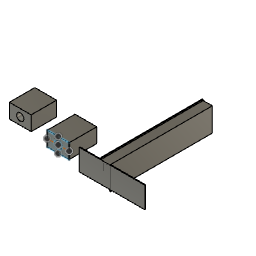
WhiteBoardMount v10 (Autodesk Fusion 360 design; units mm, degrees)
Autodesk Fusion 360 part; units mm, degrees
sketch "Sketch1" plane through (0, 0, 0) normal (0, 1, 0) x (1, 0, 0) in component "Mount"
  line L0 (0, 0) -> (-4.6, 0)
  line L1 (0, 0) -> (0, 30)
  line L2 (0, 30) -> (2, 30)
  line L3 (2, 30) -> (2, -4)
  line L4 (-4.6, 0) -> (-4.6, 10)
  line L5 (-4.6, 10) -> (-6.6, 10)
  line L6 (-6.6, 10) -> (-6.6, 0)
  line L7 (-6.6, 0) -> (-11.6, 0)
  line L8 (-11.6, 0) -> (-11.6, -4)
  line L9 (-11.6, -4) -> (2, -4)
  line L10 (-11.6, -4) -> (-10.6, -4)
  line L11 (-10.6, -4) -> (-10.6, -4)
  line L12 (-10.6, -4) -> (-11.6, -4)
  line L13 (-11.6, -4) -> (-11.6, -4)
  line L14 (-10.6, -4) -> (-10.6, -2.5)
  line L15 (2, -2.5) -> (1, -2.5) construction
  line L16 (-10.6, -2.5) -> (2, -2.5)
  line L17 (50.1972, -2.5) -> (-40, -2.5)
  line L18 (-40, -2.5) -> (-40, 0)
  line L19 (-40, 0) -> (50.1972, 0)
  line L20 (50.1972, 0) -> (50.1972, -2.5)
  line L21 (50, 23.4656) -> (-40, 23.4656)
  line L22 (-40, 23.4656) -> (-40, 21.2216)
  line L23 (-40, 21.2216) -> (50, 21.2216)
  line L24 (50, 21.2216) -> (50, 23.4656)
  dimension "d1" = 4.6
  dimension "d2" = 30
  dimension "d3" = 2
  dimension "d4" = 34
  dimension "d5" = 2
  dimension "d6" = 10
  dimension "d7" = 10
  dimension "d8" = 5
  dimension "d9" = 4
  dimension "d14" = 1
  dimension "d15" = 1.5
  dimension "d16" = 1
  constraint coincident L0.start L1.start
  constraint horizontal L0
  constraint perpendicular L0 L1
  constraint perpendicular L1 L2
  constraint perpendicular L2 L3
  constraint perpendicular L0 L4
  constraint perpendicular L4 L5
  constraint perpendicular L5 L6
  constraint perpendicular L6 L7
  constraint perpendicular L7 L8
  constraint horizontal L10
  constraint horizontal L12
  constraint perpendicular L9 L14
  constraint coincident L3 L15.start
  constraint perpendicular L3 L15
  constraint perpendicular L3 L16
  constraint horizontal L17
  constraint vertical L18
  constraint horizontal L19
  constraint vertical L20
  constraint horizontal L21
  constraint vertical L22
  constraint horizontal L23
  constraint vertical L24
  measures "d1" distance of L0.start L0.end
  measures "d2" distance of L0.start L1.end
  measures "d3" distance of L1.end L2.end
  measures "d4" distance of L2.end L3.end
  measures "d5" distance of L4.end L5.end
  measures "d6" distance of L0.end L4.end
  measures "d7" distance of L5.end L6.end
  measures "d8" distance of L6.end L7.end
  measures "d9" distance of L7.end L8.end
  measures "d14" distance of L8.end L10.end
  measures "d15" distance of L10.end L14.end
  measures "d16" distance of L15.start L15.end
extrude "Extrude1" add sketch "Sketch1" along normal blind 140 contours L0 L3 L7 L8 L16 L17 L19 | L1 L3 L19 L23 | L4 L5 L6 L19 | L1 L3 L21 L23 | L1 L2 L3 L21 | L8 L9 L10 L12 L14 L17 makes body 1 in component "Mount"
form "Form1" [no effect] in component "Mount"
fillet "Fillet2" radius 1 tangency weight 0.82684 3 edges at (-4.6, 70, -10) (0, 70, -30) (-6.6, 70, -10) on bodies 1 in component "Mount"
sketch "Sketch1 (2)" plane through (0, 0, 0) normal (0, 1, 0) x (1, 0, 0) in component "Draining BoardMount Back right"
  line L0 (-85, 0) -> (-55, 0)
  line L1 (-55, 0) -> (-55, 20)
  line L2 (-55, 20) -> (-85, 20)
  line L3 (-85, 20) -> (-85, 0)
  line L4 (-70, 0) -> (-70, 20) construction
  line L5 (-55, 10) -> (-85, 10) construction
  circle A0 centre (-70, 10) radius 5
  point P0 (-85, 10)
  point P1 (-55, 10)
  point P2 (-70, 0)
  point P3 (-70, 20)
  dimension "d21" = 30
  dimension "d22" = 20
  dimension "d23" = 55
  dimension "d24" = 10
  constraint horizontal L0
  constraint vertical L1
  constraint horizontal L2
  constraint vertical L3
  constraint midpoint L3 P0
  constraint midpoint L1 P1
  constraint midpoint L0 P2
  constraint midpoint L2 P3
  constraint coincident P2 L4.start
  constraint coincident P3 L4.end
  constraint coincident P1 L5.start
  constraint coincident P0 L5.end
  constraint midpoint L5 A0.centre
  measures "d21" distance of L0.start L0.end
  measures "d22" distance of L0.start L2.end
  measures "d23" distance of origin L0.end
  measures "d24" diameter of A0
extrude "Extrude1'" add sketch "Sketch1 (2)" along normal blind 38 separate body contours L0 L1 L2 L3 | A0 makes body 2 in component "Draining BoardMount Back right"
extrude "Extrude2" cut sketch "Sketch1 (2)" along normal blind 8 contours A0 bodies 2 in component "Draining BoardMount Back right"
sketch "Sketch1 (3)" plane through (0, 0, 0) normal (0, 1, 0) x (1, 0, 0) in component "Draining BoardMount Front right"
  line L0 (-85, 0) -> (-55, 0)
  line L1 (-55, 0) -> (-55, 20)
  line L2 (-55, 20) -> (-85, 20)
  line L3 (-85, 20) -> (-85, 0)
  line L4 (-70, 0) -> (-70, 20) construction
  line L5 (-55, 10) -> (-85, 10) construction
  circle A0 centre (-70, 10) radius 5
  point P0 (-85, 10)
  point P1 (-55, 10)
  point P2 (-70, 0)
  point P3 (-70, 20)
  dimension "d21_1" = 30
  dimension "d22_1" = 20
  dimension "d23_1" = 55
  dimension "d24_1" = 10
  constraint horizontal L0
  constraint vertical L1
  constraint horizontal L2
  constraint vertical L3
  constraint midpoint L3 P0
  constraint midpoint L1 P1
  constraint midpoint L0 P2
  constraint midpoint L2 P3
  constraint coincident P2 L4.start
  constraint coincident P3 L4.end
  constraint coincident P1 L5.start
  constraint coincident P0 L5.end
  constraint midpoint L5 A0.centre
  measures "d21_1" distance of L0.start L0.end
  measures "d22_1" distance of L0.start L2.end
  measures "d23_1" distance of origin L0.end
  measures "d24_1" diameter of A0
extrude "Extrude1''" add sketch "Sketch1 (3)" along normal blind 35 separate body contours L0 L1 L2 L3 | A0 makes body 3 in component "Draining BoardMount Front right"
extrude "Extrude2'" cut sketch "Sketch1 (3)" along normal blind 8 contours A0 bodies 3 in component "Draining BoardMount Front right"
extrude "Extrude3" add sketch "Sketch1" against normal blind 1 contours L0 L3 L7 L8 L16 L17 L19 | L1 L21 L22 L23 | L1 L3 L21 L23 | L3 L17 L19 L20 | L3 L21 L23 L24 | L8 L17 L18 L19 bodies 1 in component "Mount"
sketch "Sketch2" plane through (0, -1, 0) normal (0, -1, 0) x (1, 0, 0) in component "Mount"
  line L0 (-40, 0) -> (50.1972, 0)
  line L1 (50.1972, 0) -> (50.1972, 2.5)
  line L2 (50.1972, 2.5) -> (-40, 2.5)
  line L3 (-40, 2.5) -> (-40, 0)
  line L4 (-40, 2.5) -> (50.1972, 2.5)
  line L5 (50.1972, 2.5) -> (50.1972, -26.7747)
  line L6 (50.1972, -26.7747) -> (-40, -26.7747)
  line L7 (-40, -26.7747) -> (-40, 2.5)
  constraint horizontal L4
  constraint vertical L5
  constraint horizontal L6
  constraint vertical L7
  constraint coincident L2.end L3.start
extrude "Extrude4" add sketch "Sketch2" against normal blind 1 contours L0 L5 L6 L7 bodies 1 in component "Mount"
component "Mount" placed x (1, 0, 0) y (0, 1, 0) z (0, 0, 1) at (0, 0, 0)
component "Draining BoardMount Back right" placed x (1, 0, 0) y (0, 1, 0) z (0, 0, 1) at (0, 0, 0)
component "Draining BoardMount Front right" placed x (1, 0, 0) y (0, 1, 0) z (0, 0, 1) at (-52.2813, 0, 7.0883)
equation "d4 = d2 + d3 + 2 mm"
equation "d5 = d3"
equation "d7 = d6"
equation "d9 = d3 + 2 mm"
named bodies: "Draining BoardMount Back right"
